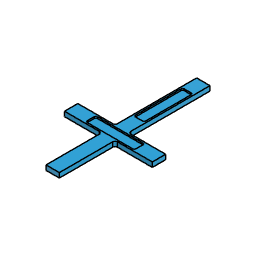
シロコ_ヘアピン_mk2 v12 (Autodesk Fusion 360 design; units mm, degrees)
Autodesk Fusion 360 part; units mm, degrees
sketch "スケッチ1" plane through (0, 0, 0) normal (0, 0, 1) x (1, 0, 0) in component "main"
  line L0 (0, 0) -> (0, 8.5)
  line L1 (0, 0) -> (56, 0) construction
  line L2 (0, 8.5) -> (56, 8.5) construction
  line L3 (56, 8.5) -> (56, 0)
  line L4 (28, 8.5) -> (28, 60.5) construction
  line L5 (28, 0) -> (28, -35.5) construction
  line L6 (23.75, 60.5) -> (32.25, 60.5)
  line L7 (23.75, 60.5) -> (23.75, 8.5)
  line L8 (32.25, 60.5) -> (32.25, 8.5)
  line L9 (23.75, -35.5) -> (32.25, -35.5)
  line L10 (23.75, -35.5) -> (23.75, 0)
  line L11 (32.25, -35.5) -> (32.25, 0)
  line L12 (0, 8.5) -> (23.75, 8.5)
  line L13 (32.25, 8.5) -> (56, 8.5)
  line L14 (0, 0) -> (23.75, 0)
  line L15 (32.25, 0) -> (56, 0)
  line L16 (28, 8.5) -> (28, 0) construction
  line L17 (0, 4.25) -> (56, 4.25) construction
  line L18 (12.5, 7.5) -> (43.5, 7.5)
  line L19 (43.5, 7.5) -> (43.5, 1)
  line L20 (43.5, 1) -> (12.5, 1)
  line L21 (12.5, 1) -> (12.5, 7.5)
  line L22 (24.75, 50.5) -> (31.25, 50.5)
  line L23 (31.25, 50.5) -> (31.25, 19.5)
  line L24 (31.25, 19.5) -> (24.75, 19.5)
  line L25 (24.75, 19.5) -> (24.75, 50.5)
  dimension "d1" = 8.5
  dimension "d2" = 56
  dimension "d3" = 52
  dimension "d4" = 96
  dimension "d5" = 8.5
  dimension "d6" = 8.5
  dimension "d15" = 31
  dimension "d16" = 6.5
  dimension "d25" = 6.5
  dimension "d26" = 31
  dimension "d27" = 10
  constraint coincident L0.start L1.start
  constraint vertical L0
  constraint perpendicular L0 L1
  constraint perpendicular L0 L2
  constraint perpendicular L1 L3
  constraint midpoint L2 L4.start
  constraint perpendicular L2 L4
  constraint midpoint L1 L5.start
  constraint perpendicular L1 L5
  constraint perpendicular L4 L6
  constraint midpoint L4.end L6
  constraint coincident L2 L7.end
  constraint perpendicular L2 L7
  constraint coincident L2 L8.end
  constraint perpendicular L2 L8
  constraint perpendicular L4 L9
  constraint midpoint L5.end L9
  constraint coincident L1 L10.end
  constraint perpendicular L1 L10
  constraint coincident L1 L11.end
  constraint perpendicular L1 L11
  constraint midpoint L0 L17.start
  constraint midpoint L3 L17.end
  constraint horizontal L18
  constraint vertical L19
  constraint horizontal L20
  constraint vertical L21
  constraint symmetric L17 L18 L20
  constraint symmetric L16 L19 L21
  constraint horizontal L22
  constraint vertical L23
  constraint horizontal L24
  constraint vertical L25
  constraint symmetric L4 L23 L25
  measures "d1" distance of L0.start L0.end
  measures "d2" distance of L0.start L1.end
  measures "d3" distance of L4.start L4.end
  measures "d4" distance of L4.end L5.end
  measures "d5" distance of L6.start L6.end
  measures "d6" distance of L9.start L9.end
  measures "d15" distance of L18.start L18.end
  measures "d16" distance of L18.start L20.end
  measures "d25" distance of L22.start L22.end
  measures "d26" distance of L22.start L24.end
  measures "d27" distance of L4.end L22
extrude "押し出し7" add sketch "スケッチ1" against normal blind 3 contours L0 L3 L6 L7 L8 L9 L10 L11 L12 L13 L14 L15 | L18 L19 L20 L21 | L22 L23 L24 L25 in component "main"
extrude "押し出し8" cut sketch "スケッチ1" against normal blind 1 contours L18 L19 L20 L21 | L22 L23 L24 L25 in component "main"
move_body "移動3" bodies 1 to x (1, 0, 0) y (0, 1, 0) z (0, 0, 1) at (0, 0, 3) in component "main"
fillet "フィレット8" radius 1 4 edges at (12.5, 7.5, 2.5) (43.5, 7.5, 2.5) (43.5, 1, 2.5) (12.5, 1, 2.5) in component "main"
fillet "フィレット9" radius 1 4 edges at (31.25, 19.5, 2.5) (31.25, 50.5, 2.5) (24.75, 50.5, 2.5) (24.75, 19.5, 2.5) in component "main"
fillet "フィレット10" radius 1.5 4 edges at (32.25, 8.5, 1.5) (23.75, 8.5, 1.5) (23.75, 0, 1.5) (32.25, 0, 1.5) in component "main"
component "main" placed x (1, 0, 0) y (0, 1, 0) z (0, 0, 1) at (0, 0, 0)
